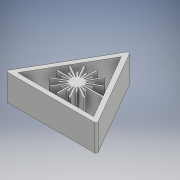
# Autodesk Inventor part: Logo Laser
Saved by Autodesk Inventor 2017 (Build 210142000, 142)
## iProperties
Part Number: Logo Laser
Material: Générique
Document SubType Name: Modeling
Designer: Adrien MARY
Density: 1 g/cm^3
Appearance: Par défaut
Stock Number: 1410-01-07
Project: 1410 LaserShow
Author: Adrien MARY
Autodesk Inventor part; units mm, degrees
ref_plane "YZ Plane" through (0, 0, 0) normal (1, 0, 0) x (0, 1, 0)
ref_plane "XZ Plane" through (0, 0, 0) normal (0, 1, 0) x (-1, 0, 0)
ref_plane "XY Plane" through (0, 0, 0) normal (0, 0, 1) x (1, 0, 0)
sketch "Esquisse3" plane through (0, 0, 0) normal (0, 0, 1) x (1, 0, 0)
  line L0 (-97.75, 106.7859) -> (105.7088, 106.7859) construction
  line L1 (105.7088, 106.7859) -> (105.7088, -86.5) construction
  line L2 (105.7088, -86.5) -> (-97.75, -86.5) construction
  line L3 (-97.75, -86.5) -> (-97.75, 106.7859) construction
  circle A0 centre (0, 0) radius 11.5
  line L4 (-1.5, 0) -> (1.5, 0)
  line L5 (1.5, 0) -> (1.5, 38)
  line L6 (1.5, 38) -> (-1.5, 38)
  line L7 (-1.5, 38) -> (-1.5, 0)
  circle A1 centre (0, 0) radius 11.5 construction
  line L8 (-1.299, -0.75) -> (1.299, 0.75)
  line L9 (1.299, 0.75) -> (-17.701, 33.659)
  line L10 (-17.701, 33.659) -> (-20.299, 32.159)
  line L11 (-20.299, 32.159) -> (-1.299, -0.75)
  circle A2 centre (0, 0) radius 11.5 construction
  line L12 (-0.75, -1.299) -> (0.75, 1.299)
  line L13 (0.75, 1.299) -> (-32.159, 20.299)
  line L14 (-32.159, 20.299) -> (-33.659, 17.701)
  line L15 (-33.659, 17.701) -> (-0.75, -1.299)
  circle A3 centre (0, 0) radius 11.5 construction
  line L16 (0, -1.5) -> (0, 1.5)
  line L17 (0, 1.5) -> (-38, 1.5)
  line L18 (-38, 1.5) -> (-38, -1.5)
  line L19 (-38, -1.5) -> (0, -1.5)
  line L20 (-17.701, -33.659) -> (1.299, -0.75)
  line L21 (-0.75, -1.299) -> (0.75, 1.299)
  line L22 (-1.299, 0.75) -> (-20.299, -32.159)
  line L23 (-33.659, -17.701) -> (-32.159, -20.299)
  line L24 (-0.75, 1.299) -> (-33.659, -17.701)
  line L25 (-38, 1.5) -> (-38, -1.5)
  line L26 (0, 1.5) -> (-38, 1.5)
  line L27 (-33.659, 17.701) -> (-0.75, -1.299)
  line L28 (0.75, 1.299) -> (-32.159, 20.299)
  line L29 (-32.159, 20.299) -> (-33.659, 17.701)
  line L30 (-20.299, -32.159) -> (-17.701, -33.659)
  line L31 (-38, -1.5) -> (0, -1.5)
  line L32 (-32.159, -20.299) -> (0.75, -1.299)
  line L33 (1.299, -0.75) -> (-1.299, 0.75)
  line L34 (0.75, -1.299) -> (-0.75, 1.299)
  line L35 (0, -1.5) -> (0, 1.5)
  line L36 (20.299, -32.159) -> (1.299, 0.75)
  line L37 (0.75, -1.299) -> (-0.75, 1.299)
  line L38 (-1.299, -0.75) -> (17.701, -33.659)
  line L39 (-1.5, -38) -> (1.5, -38)
  line L40 (-1.5, 0) -> (-1.5, -38)
  line L41 (-20.299, -32.159) -> (-17.701, -33.659)
  line L42 (-1.299, 0.75) -> (-20.299, -32.159)
  line L43 (-32.159, -20.299) -> (0.75, -1.299)
  line L44 (-0.75, 1.299) -> (-33.659, -17.701)
  line L45 (-33.659, -17.701) -> (-32.159, -20.299)
  line L46 (17.701, -33.659) -> (20.299, -32.159)
  line L47 (-17.701, -33.659) -> (1.299, -0.75)
  line L48 (1.5, -38) -> (1.5, 0)
  line L49 (1.299, 0.75) -> (-1.299, -0.75)
  line L50 (1.5, 0) -> (-1.5, 0)
  line L51 (1.299, -0.75) -> (-1.299, 0.75)
  line L52 (38, 1.5) -> (0, 1.5)
  line L53 (1.5, 0) -> (-1.5, 0)
  line L54 (0, -1.5) -> (38, -1.5)
  line L55 (32.159, -20.299) -> (33.659, -17.701)
  line L56 (-0.75, -1.299) -> (32.159, -20.299)
  line L57 (17.701, -33.659) -> (20.299, -32.159)
  line L58 (-1.299, -0.75) -> (17.701, -33.659)
  line L59 (1.5, -38) -> (1.5, 0)
  line L60 (-1.5, 0) -> (-1.5, -38)
  line L61 (-1.5, -38) -> (1.5, -38)
  line L62 (38, -1.5) -> (38, 1.5)
  line L63 (20.299, -32.159) -> (1.299, 0.75)
  line L64 (33.659, -17.701) -> (0.75, 1.299)
  line L65 (0, 1.5) -> (0, -1.5)
  line L66 (0.75, 1.299) -> (-0.75, -1.299)
  line L67 (1.299, 0.75) -> (-1.299, -0.75)
  line L68 (17.701, 33.659) -> (-1.299, 0.75)
  line L69 (0.75, 1.299) -> (-0.75, -1.299)
  line L70 (1.299, -0.75) -> (20.299, 32.159)
  line L71 (33.659, 17.701) -> (32.159, 20.299)
  line L72 (0.75, -1.299) -> (33.659, 17.701)
  line L73 (38, -1.5) -> (38, 1.5)
  line L74 (0, -1.5) -> (38, -1.5)
  line L75 (33.659, -17.701) -> (0.75, 1.299)
  line L76 (-0.75, -1.299) -> (32.159, -20.299)
  line L77 (32.159, -20.299) -> (33.659, -17.701)
  line L78 (20.299, 32.159) -> (17.701, 33.659)
  line L79 (38, 1.5) -> (0, 1.5)
  line L80 (32.159, 20.299) -> (-0.75, 1.299)
  line L81 (-1.299, 0.75) -> (1.299, -0.75)
  line L82 (-0.75, 1.299) -> (0.75, -1.299)
  line L83 (0, 1.5) -> (0, -1.5)
  line L84 (-20.299, 32.159) -> (-1.299, -0.75)
  line L85 (-0.75, 1.299) -> (0.75, -1.299)
  line L86 (1.299, 0.75) -> (-17.701, 33.659)
  line L87 (1.5, 38) -> (-1.5, 38)
  line L88 (1.5, 0) -> (1.5, 38)
  line L89 (20.299, 32.159) -> (17.701, 33.659)
  line L90 (1.299, -0.75) -> (20.299, 32.159)
  line L91 (32.159, 20.299) -> (-0.75, 1.299)
  line L92 (0.75, -1.299) -> (33.659, 17.701)
  line L93 (33.659, 17.701) -> (32.159, 20.299)
  line L94 (-17.701, 33.659) -> (-20.299, 32.159)
  line L95 (17.701, 33.659) -> (-1.299, 0.75)
  line L96 (-1.5, 38) -> (-1.5, 0)
  line L97 (-1.299, -0.75) -> (1.299, 0.75)
  line L98 (-1.5, 0) -> (1.5, 0)
  line L99 (-1.299, 0.75) -> (1.299, -0.75)
  line L100 (-3.6093, 7.914) -> (-7.1789, 24.0155)
  line L101 (-7.1789, 24.0155) -> (-4.25, 24.6648)
  line L102 (-4.25, 24.6648) -> (-0.6804, 8.5633)
  line L103 (-0.6804, 8.5633) -> (-3.6093, 7.914)
  line L104 (-3.6093, 7.914) -> (-4.25, 24.6648) construction
  line L105 (-7.1789, 24.0155) -> (-0.6804, 8.5633) construction
  line L106 (-4.8709, 7.0758) -> (-7.0827, 5.0491)
  line L107 (-16.013, 19.2353) -> (-4.8709, 7.0758)
  line L108 (-7.0827, 5.0491) -> (-18.2248, 17.2086)
  line L109 (-7.7562, 3.6924) -> (-8.6583, 0.8313)
  line L110 (-23.4853, 8.6518) -> (-7.7562, 3.6924)
  line L111 (-8.6583, 0.8313) -> (-24.3874, 5.7906)
  line L112 (-8.5633, -0.6804) -> (-7.914, -3.6093)
  line L113 (-24.6648, -4.25) -> (-8.5633, -0.6804)
  line L114 (-7.914, -3.6093) -> (-24.0155, -7.1789)
  line L115 (-18.2248, 17.2086) -> (-16.013, 19.2353)
  line L116 (-24.3874, 5.7906) -> (-23.4853, 8.6518)
  line L117 (-24.0155, -7.1789) -> (-24.6648, -4.25)
  line L118 (-0.8313, -8.6583) -> (-5.7906, -24.3874)
  line L119 (-8.6518, -23.4853) -> (-3.6924, -7.7562)
  line L120 (-5.7906, -24.3874) -> (-8.6518, -23.4853)
  line L121 (-3.6924, -7.7562) -> (-0.8313, -8.6583)
  line L122 (-17.2086, -18.2248) -> (-19.2353, -16.013)
  line L123 (-5.0491, -7.0827) -> (-17.2086, -18.2248)
  line L124 (-19.2353, -16.013) -> (-7.0758, -4.8709)
  line L125 (-7.914, -3.6093) -> (-24.0155, -7.1789)
  line L126 (-24.0155, -7.1789) -> (-24.6648, -4.25)
  line L127 (-24.6648, -4.25) -> (-8.5633, -0.6804)
  line L128 (-7.0758, -4.8709) -> (-5.0491, -7.0827)
  line L129 (-7.7562, 3.6924) -> (-8.6583, 0.8313)
  line L130 (-8.6583, 0.8313) -> (-24.3874, 5.7906)
  line L131 (-23.4853, 8.6518) -> (-7.7562, 3.6924)
  line L132 (-8.5633, -0.6804) -> (-7.914, -3.6093)
  line L133 (-24.3874, 5.7906) -> (-23.4853, 8.6518)
  line L134 (7.0827, -5.0491) -> (18.2248, -17.2086)
  line L135 (16.013, -19.2353) -> (4.8709, -7.0758)
  line L136 (18.2248, -17.2086) -> (16.013, -19.2353)
  line L137 (4.8709, -7.0758) -> (7.0827, -5.0491)
  line L138 (7.1789, -24.0155) -> (4.25, -24.6648)
  line L139 (3.6093, -7.914) -> (7.1789, -24.0155)
  line L140 (4.25, -24.6648) -> (0.6804, -8.5633)
  line L141 (-0.8313, -8.6583) -> (-5.7906, -24.3874)
  line L142 (-5.7906, -24.3874) -> (-8.6518, -23.4853)
  line L143 (-8.6518, -23.4853) -> (-3.6924, -7.7562)
  line L144 (0.6804, -8.5633) -> (3.6093, -7.914)
  line L145 (-7.0758, -4.8709) -> (-5.0491, -7.0827)
  line L146 (-5.0491, -7.0827) -> (-17.2086, -18.2248)
  line L147 (-19.2353, -16.013) -> (-7.0758, -4.8709)
  line L148 (-3.6924, -7.7562) -> (-0.8313, -8.6583)
  line L149 (-17.2086, -18.2248) -> (-19.2353, -16.013)
  line L150 (7.914, 3.6093) -> (24.0155, 7.1789)
  line L151 (24.6648, 4.25) -> (8.5633, 0.6804)
  line L152 (24.0155, 7.1789) -> (24.6648, 4.25)
  line L153 (8.5633, 0.6804) -> (7.914, 3.6093)
  line L154 (24.3874, -5.7906) -> (23.4853, -8.6518)
  line L155 (8.6583, -0.8313) -> (24.3874, -5.7906)
  line L156 (23.4853, -8.6518) -> (7.7562, -3.6924)
  line L157 (7.0827, -5.0491) -> (18.2248, -17.2086)
  line L158 (18.2248, -17.2086) -> (16.013, -19.2353)
  line L159 (16.013, -19.2353) -> (4.8709, -7.0758)
  line L160 (7.7562, -3.6924) -> (8.6583, -0.8313)
  line L161 (0.6804, -8.5633) -> (3.6093, -7.914)
  line L162 (3.6093, -7.914) -> (7.1789, -24.0155)
  line L163 (4.25, -24.6648) -> (0.6804, -8.5633)
  line L164 (4.8709, -7.0758) -> (7.0827, -5.0491)
  line L165 (7.1789, -24.0155) -> (4.25, -24.6648)
  line L166 (0.8313, 8.6583) -> (5.7906, 24.3874)
  line L167 (8.6518, 23.4853) -> (3.6924, 7.7562)
  line L168 (5.7906, 24.3874) -> (8.6518, 23.4853)
  line L169 (3.6924, 7.7562) -> (0.8313, 8.6583)
  line L170 (17.2086, 18.2248) -> (19.2353, 16.013)
  line L171 (5.0491, 7.0827) -> (17.2086, 18.2248)
  line L172 (19.2353, 16.013) -> (7.0758, 4.8709)
  line L173 (7.914, 3.6093) -> (24.0155, 7.1789)
  line L174 (24.0155, 7.1789) -> (24.6648, 4.25)
  line L175 (24.6648, 4.25) -> (8.5633, 0.6804)
  line L176 (7.0758, 4.8709) -> (5.0491, 7.0827)
  line L177 (7.7562, -3.6924) -> (8.6583, -0.8313)
  line L178 (8.6583, -0.8313) -> (24.3874, -5.7906)
  line L179 (23.4853, -8.6518) -> (7.7562, -3.6924)
  line L180 (8.5633, 0.6804) -> (7.914, 3.6093)
  line L181 (24.3874, -5.7906) -> (23.4853, -8.6518)
  line L182 (-7.0827, 5.0491) -> (-18.2248, 17.2086)
  line L183 (-16.013, 19.2353) -> (-4.8709, 7.0758)
  line L184 (-18.2248, 17.2086) -> (-16.013, 19.2353)
  line L185 (-4.8709, 7.0758) -> (-7.0827, 5.0491)
  line L186 (-7.1789, 24.0155) -> (-4.25, 24.6648)
  line L187 (-3.6093, 7.914) -> (-7.1789, 24.0155)
  line L188 (-4.25, 24.6648) -> (-0.6804, 8.5633)
  line L189 (0.8313, 8.6583) -> (5.7906, 24.3874)
  line L190 (5.7906, 24.3874) -> (8.6518, 23.4853)
  line L191 (8.6518, 23.4853) -> (3.6924, 7.7562)
  line L192 (-0.6804, 8.5633) -> (-3.6093, 7.914)
  line L193 (7.0758, 4.8709) -> (5.0491, 7.0827)
  line L194 (5.0491, 7.0827) -> (17.2086, 18.2248)
  line L195 (19.2353, 16.013) -> (7.0758, 4.8709)
  line L196 (3.6924, 7.7562) -> (0.8313, 8.6583)
  line L197 (17.2086, 18.2248) -> (19.2353, 16.013)
  line L198 (-71.285, -41.126) -> (72.8576, -41.126)
  line L199 (72.8576, -41.126) -> (0.8283, 83.2506)
  line L200 (0.8283, 83.2506) -> (-71.285, -41.126)
  line L201 (-81.5097, -50.0167) -> (83.0763, -50.0167)
  line L202 (85.6724, -45.5133) -> (3.4273, 96.5034)
  line L203 (-1.7641, 96.5048) -> (-84.105, -45.512)
  arc A4 (-84.105, -45.512) -> (-81.5097, -50.0167) centre (-81.5097, -47.0167) ccw
  arc A5 (83.0763, -50.0167) -> (85.6724, -45.5133) centre (83.0763, -47.0167) ccw
  arc A6 (3.4273, 96.5034) -> (-1.7641, 96.5048) centre (0.8313, 95) ccw
  line L204 (34.3249, -1.5) -> (55, -1.5)
  line L205 (55, -1.5) -> (55, 1.5)
  line L206 (55, 1.5) -> (34.3249, 1.5)
  line L207 (34.3249, 1.5) -> (34.3249, -1.5)
  point P0 (0, 38)
  point P1 (-19, 32.909)
  point P2 (-32.909, 19)
  point P3 (-38, 0)
  point P4 (-32.909, -19)
  point P5 (-38, 0)
  point P6 (-32.909, 19)
  point P7 (-141.3543, -31.2611)
  point P8 (-19, -32.909)
  point P9 (0, -38)
  point P10 (-19, -32.909)
  point P11 (-32.909, -19)
  point P12 (-43.6043, -138.0469)
  point P13 (19, -32.909)
  point P14 (32.909, -19)
  point P15 (19, -32.909)
  point P16 (0, -38)
  point P17 (97.75, -106.7859)
  point P18 (38, 0)
  point P19 (32.909, 19)
  point P20 (38, 0)
  point P21 (32.909, -19)
  point P22 (141.3543, 31.2611)
  point P23 (19, 32.909)
  point P24 (0, 38)
  point P25 (19, 32.909)
  point P26 (32.909, 19)
  point P27 (43.6043, 138.0469)
  point P28 (-19, 32.909)
  point P29 (-3.9296, 16.2894)
  dimension "d116" = 203.4588
  dimension "d120" = 193.2859
  dimension "d121" = 97.75
  dimension "d122" = 86.5
  dimension "d124" = 23
  dimension "d125" = 3
  dimension "d128" = 38
  dimension "d133" = 90
  dimension "d138" = 360
  dimension "d143" = 3
  dimension "d155" = 25
  dimension "d157" = 12.5
  dimension "d162" = 2.75
  dimension "d165" = 90
  dimension "d170" = 360
  dimension "d179" = 3
  constraints: 408 end point, 51 coincident, 7 centre point, 6 parallel, 6 point on circle, 6 tangent, 4 midpoint, 4 perpendicular, 3 horizontal, 2 equal radius, 2 point on line, 1 vertical alignment, 551 other
  measures "d116" distance of L1.end L2.end
  measures "d120" distance of L0.end L1.end
  measures "d121" distance from line of point (0, 0) L3
  measures "d122" distance from line of L2 point (0, 0)
  measures "d124" diameter of A0
  measures "d125" distance of L5.end L6.end
  measures "d128" distance from line of point (0, 0) L6
  measures "d143" distance between parallel lines of L102 L100
  measures "d155" distance from line of point (0, 0) L101
  measures "d157" angle of L7 L102
  measures "d162" distance from line of L7 L101.end
  measures "d179" radius of A4
extrude "Extrusion3" add sketch "Esquisse3" along normal blind 50 contours A0 L54 L155 L160 L64 L72 L52 L153 L151 | A0 L151 L52 L207 L54 | L151 L153 L52 A0 | A0 L52 L151 | A0 L155 L54 | L52 L153 L72 L150 A0 | A0 L150 L152 L151 L52 | L155 L154 L156 L64 A0 | A0 L64 L160 L54 L155 | L54 L160 L155 | L207 L52 L62 L54 | L150 L72 A0 | L52 L72 L153 | L64 L156 A0 | A0 L156 L160 L64 | L160 L64 L54 | L62 L206 L199 L204 | L72 L150 L153 L52 L70 L80 L176 L172 A0 | A0 L172 L80 L71 L72 | L72 L153 L150 | L72 L64 L70 L52 | L156 L64 L55 L56 A0 | A0 L56 L134 L137 L36 L54 L64 L160 L156 | L54 L36 L72 L64 | L199 L206 L205 L204 | L172 L176 L80 A0 | A0 L80 L172 | L70 L64 L5 L52 | L52 L5 L80 L70 | L72 L36 L70 L64 | A0 L134 L56 | L54 L48 L72 L36 | L36 L56 L48 L54 | L80 L176 L70 L171 A0 | A0 L171 L170 L172 L80 | L52 L9 L80 L5 | L5 L64 L9 L52 | L70 L36 L5 L64 | L80 L5 L68 L169 L167 A0 L70 L171 L176 | L70 L176 L80 | L72 L48 L70 L36 | L134 L136 L135 L36 A0 | A0 L36 L137 L56 L134 | L56 L137 L134 | L56 L137 L36 | L36 L137 L135 A0 L38 L139 L144 L48 L56 | L54 L20 L72 L48 | L48 L56 L20 L54 | L171 L70 A0 | L5 L36 L9 L64 | L80 L9 L68 L5 | L52 L13 L80 L9 | L9 L64 L13 L52 | L70 L48 L5 L36 | L176 L171 L70 | L72 L20 L70 L48 | L36 L135 A0 | A0 L135 L137 L36 | L48 L38 L20 L56 | L54 L32 L72 L20 | L20 L56 L32 L54 | A0 L167 L68 L78 L70 | L5 L4 L8 L36 | L9 L8 L12 L64 | L68 L9 L7 L103 L102 A0 L5 L166 L169 | L5 L169 L68 | L80 L13 L68 L9 | L52 L17 L80 L13 | L13 L12 L16 L52 | L70 L33 L4 L48 | L72 L34 L33 L20 | L135 L36 L46 L38 A0 | L48 L144 L140 A0 L40 L118 L121 L20 L38 | L38 L144 L48 | L20 L38 L32 L56 | L54 L16 L34 L32 | L32 L56 L19 L54 | L167 L169 L68 A0 | A0 L68 L167 | L169 L166 L5 | L5 L166 A0 L68 L169 | L68 L13 L7 L9 | L80 L17 L68 L13 | L16 L34 L80 L17 | A0 L139 L38 | L20 L40 L32 L38 | L144 L139 L38 | L38 L139 A0 L48 L144 | L48 A0 L140 L144 | L32 L38 L19 L56 | L19 L56 L12 L16 | A0 L166 L168 L167 L68 | L8 L11 L40 L4 | L12 L15 L38 L8 | L4 L7 L22 L33 | L33 L68 L24 L34 | L5 A0 L166 | L9 L103 L7 | L7 L13 L11 L106 L107 A0 L9 L100 L103 | L68 L17 L7 L13 | L80 L24 L68 L17 | L139 L138 L140 L48 A0 | L40 L121 L20 | L20 L121 L119 A0 L22 L123 L128 L32 L40 | L32 L40 L19 L38 | L48 L140 A0 | L19 L38 L15 L56 | L40 L11 L22 L7 | L38 L15 L40 L11 | L22 L7 L24 L68 | A0 L102 L7 L6 L5 | L103 L9 L100 A0 L7 | L7 A0 L102 L103 | L7 L17 L11 L13 | L103 L100 L9 | L68 L24 L7 L17 | L121 L40 L118 A0 L20 | L20 A0 L119 L121 | L32 L22 L19 L40 | L121 L118 L40 | L19 L40 L15 L38 | L140 L48 L39 L40 A0 | L22 L11 L24 L7 | L40 L15 L22 L11 | A0 L7 L102 | A0 L100 L101 L102 L7 | L7 L24 L11 L17 | L13 L106 L11 | L11 L17 L15 L109 L110 A0 L13 L108 L106 | L9 A0 L100 | L20 L119 A0 | A0 L118 L120 L119 L20 | L32 L128 L124 A0 L24 L114 L112 L19 L22 | L22 L128 L32 | L19 L22 L15 L40 | L40 A0 L118 | L22 L15 L24 L11 | L11 L24 L15 L17 | L106 L13 L108 A0 L11 | L11 A0 L107 L106 | L106 L108 L13 | A0 L107 L11 L10 L9 | L119 L20 L30 L22 A0 | L19 L24 L15 L22 | L128 L123 L22 | L22 L123 A0 L32 L128 | L32 A0 L124 L128 | L17 L109 L15 | L15 L24 L19 L112 L113 A0 L17 L111 L109 | L11 L107 A0 | A0 L108 L115 L107 L11 | L13 A0 L108 | A0 L123 L22 | L24 L112 L19 | L32 L124 A0 | A0 L123 L122 L124 L32 | L109 L17 L111 A0 L15 | L15 A0 L110 L109 | L109 L111 L17 | A0 L110 L15 L14 L13 | L112 L24 L114 A0 L19 | L19 A0 L113 L112 | L112 L114 L24 | L124 L32 L23 L24 A0 | L15 L110 A0 | A0 L111 L116 L110 L15 | L17 A0 L111 | L19 L113 A0 | A0 L114 L117 L113 L19 | L24 A0 L114 | A0 L113 L19 L18 L17 | A4 L203 A6 L202 A5 L201
equation "\"pi\" = 3.141593"
equation "\"nombredor\" = 1.61803"
